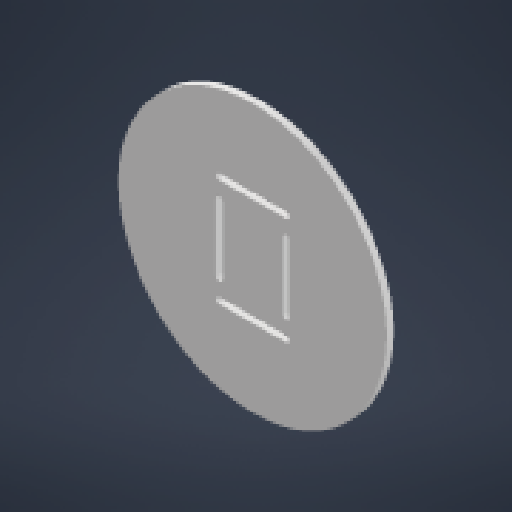
# Autodesk Inventor part: tableStandTop
Saved by Autodesk Inventor 2026.3 (Build 303398000, 398)
## iProperties
Created: 2026-06-26
Part Number: tableStandTop
Material: Generic
Document SubType Name: Modeling
Designer: frede
Density: 1 g/cm^3
Appearance: Default
Author: frede
Autodesk Inventor part; units mm, degrees
ref_plane "YZ Plane" through (0, 0, 0) normal (1, 0, 0) x (0, 1, 0)
ref_plane "XZ Plane" through (0, 0, 0) normal (0, 1, 0) x (-1, 0, 0)
ref_plane "XY Plane" through (0, 0, 0) normal (0, 0, 1) x (1, 0, 0)
sketch "Sketch1" plane through (0, 0, 0) normal (0, 0, 1) x (1, 0, 0)
  circle A0 centre (0, 0) radius 100
  arc A1 (-22.8, 25) -> (-27.2, 25) centre (-25, 25) ccw
  line L0 (-25, 25) -> (-25, -25)
  arc A2 (-27.2, -25) -> (-22.8, -25) centre (-25, -25) ccw
  line L1 (-27.2, -25) -> (-27.2, 25)
  line L2 (-22.8, 25) -> (-22.8, -25)
  arc A3 (-25, 42.2) -> (-25, 37.8) centre (-25, 40) ccw
  line L3 (-25, 40) -> (25, 40)
  arc A4 (25, 37.8) -> (25, 42.2) centre (25, 40) ccw
  line L4 (-25, 42.2) -> (25, 42.2)
  line L5 (25, 37.8) -> (-25, 37.8)
  arc A5 (25, -42.2) -> (25, -37.8) centre (25, -40) ccw
  arc A6 (-25, -37.8) -> (-25, -42.2) centre (-25, -40) ccw
  line L6 (25, -42.2) -> (-25, -42.2)
  line L7 (-25, -37.8) -> (25, -37.8)
  line L8 (25, -40) -> (-25, -40)
  arc A7 (22.8, -25) -> (27.2, -25) centre (25, -25) ccw
  line L9 (25, -25) -> (25, 25)
  line L10 (27.2, 25) -> (27.2, -25)
  line L11 (22.8, -25) -> (22.8, 25)
  arc A8 (27.2, 25) -> (22.8, 25) centre (25, 25) ccw
  dimension "d0" = 200
  dimension "d1" = 4.4
  dimension "d2" = 50
  dimension "d3" = 4.4
  dimension "d8" = 4.4
  dimension "d9" = 50
  dimension "d10" = 4.4
  dimension "d11" = 40
  dimension "d14" = 360
  constraints: 24 end point, 16 point on circle, 9 centre point, 5 coincident, 5 tangent, 1 horizontal, 1 parallel, 1 vertical, 49 other
  measures "d0" diameter of A0
  measures "d1" diameter of A1
  measures "d2" distance of L0.start L0.end
  measures "d3" diameter of A2
  measures "d8" diameter of A3
  measures "d9" distance of L3.start L3.end
  measures "d10" diameter of A4
  measures "d11" distance from line of point (0, 0) L3
extrude "Extrusion1" add sketch "Sketch1" along normal blind 5
sketch "Sketch2" plane through (0, 0, 5) normal (0, 0, 1) x (1, 0, 0)
  circle A0 centre (-63.8814, 25.501) radius 5 projected
  circle A1 centre (-63.9324, -24.499) radius 5 projected
  circle A2 centre (-25.5923, -62.865) radius 5 projected
  circle A3 centre (24.4075, -63.0086) radius 5 projected
  circle A4 centre (62.7316, -24.7238) radius 5 projected
  circle A5 centre (62.7826, 25.2761) radius 5 projected
  circle A6 centre (-25.5562, 63.7395) radius 5 projected
  circle A7 centre (24.4432, 63.4944) radius 5 projected
  circle A8 centre (24.4075, -63.0086) radius 8
  circle A9 centre (-25.5923, -62.865) radius 8
  circle A10 centre (-63.9324, -24.499) radius 8
  circle A11 centre (-63.8814, 25.501) radius 8
  circle A12 centre (-25.5562, 63.7395) radius 8
  circle A13 centre (24.4432, 63.4944) radius 8
  circle A14 centre (62.7826, 25.2761) radius 8
  circle A15 centre (62.7316, -24.7238) radius 8
  point P0 (0, 0)
  dimension "d19" = 16
  dimension "d20" = 16
  dimension "d21" = 16
  dimension "d22" = 16
  dimension "d23" = 16
  dimension "d24" = 16
  dimension "d25" = 16
  dimension "d26" = 16
  constraints: 8 centre point, 8 coincident
  measures "d19" diameter of A8
  measures "d20" diameter of A9
  measures "d21" diameter of A10
  measures "d22" diameter of A11
  measures "d23" diameter of A12
  measures "d24" diameter of A13
  measures "d25" diameter of A14
  measures "d26" diameter of A15
extrude "Extrusion2" add sketch "Sketch2" along normal blind 20
fillet "Fillet1" radius 0.5 56 edges at (-25, -27.2, 5) (-27.2, 0, 5) (-25, 27.2, 5) (-22.8, 0, 5) (-25, -27.2, 0) (-27.2, 0, 0) (-25, 27.2, 0) (-22.8, 0, 0) (25, 27.2, 5) (27.2, 0, 5) (25, -27.2, 5) (22.8, 0, 5) (25, -27.2, 0) (22.8, 0, 0) (25, 27.2, 0) (27.2, 0, 0) (-27.2, 40, 5) (0, 42.2, 5) (27.2, 40, 5) (0, 37.8, 5) (-27.2, 40, 0) (0, 42.2, 0) (27.2, 40, 0) (0, 37.8, 0) (27.2, -40, 0) (0, -42.2, 0) (-27.2, -40, 0) (0, -37.8, 0) (27.2, -40, 5) (0, -42.2, 5) (-27.2, -40, 5) (0, -37.8, 5) (54.7316, -24.7238, 25) (57.7316, -24.7238, 25) (54.7826, 25.2761, 25) (57.7826, 25.2761, 25) (16.4432, 63.4944, 25) (19.4432, 63.4944, 25) (-33.5562, 63.7395, 25) (-30.5562, 63.7395, 25) (-71.8814, 25.501, 25) (-68.8814, 25.501, 25) (-71.9324, -24.499, 25) (-68.9324, -24.499, 25) (-33.5923, -62.865, 25) (-30.5923, -62.865, 25) (16.4075, -63.0086, 25) (19.4075, -63.0086, 25) (19.4075, -63.0086, 5) (57.7316, -24.7238, 5) (57.7826, 25.2761, 5) (19.4432, 63.4944, 5) (-30.5562, 63.7395, 5) (-68.8814, 25.501, 5) (-68.9324, -24.499, 5) (-30.5923, -62.865, 5)
fillet "Fillet2" radius 3 8 edges at (-33.5923, -62.865, 5) (16.4075, -63.0086, 5) (54.7316, -24.7238, 5) (54.7826, 25.2761, 5) (16.4432, 63.4944, 5) (-33.5562, 63.7395, 5) (-71.8814, 25.501, 5) (-71.9324, -24.499, 5)
equation "\"d20\" = d19"
equation "\"d21\" = d19"
equation "\"d22\" = d19"
equation "\"d23\" = d19"
equation "\"d24\" = d19"
equation "\"d25\" = d19"
equation "\"d26\" = d19"
body "Solid1"
